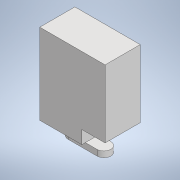
# Autodesk Inventor part: servo
Saved by Autodesk Inventor 2020 (Build 240168000, 168)
## iProperties
Created: 2022-02-17
Part Number: servo
Material: Generic
Document SubType Name: Modeling
Designer: rwte
Density: 1 g/cm^3
Appearance: Default
Author: rwte
Autodesk Inventor part; units mm, degrees
ref_plane "YZ Plane" through (0, 0, 0) normal (1, 0, 0) x (0, 1, 0)
ref_plane "XZ Plane" through (0, 0, 0) normal (0, 1, 0) x (-1, 0, 0)
ref_plane "XY Plane" through (0, 0, 0) normal (0, 0, 1) x (1, 0, 0)
sketch "Sketch1" plane through (0, 0, 0) normal (0, 0, 1) x (1, 0, 0)
  line L0 (0, 0) -> (22.5, 0)
  line L1 (22.5, 0) -> (22.5, 23.3)
  line L2 (22.5, 23.3) -> (0, 23.3)
  line L3 (0, 23.3) -> (0, 0)
  line L4 (0, 0) -> (14.5, 0)
  line L5 (14.5, 0) -> (14.5, -4.5)
  line L6 (0, -4.5) -> (0, 0)
  line L7 (0, -4.5) -> (14.5, -4.5)
  dimension "d0" = 23.3
  dimension "d1" = 22.5
  dimension "d2" = 14.5
  dimension "d3" = 4.5
  constraints: 16 end point, 3 parallel, 2 horizontal, 2 perpendicular, 1 point on line
  measures "d0" distance of L0.end L1.end
  measures "d1" distance of L1.end L2.end
  measures "d2" distance between parallel lines of L6 L5
  measures "d3" distance of L4.end L5.end
extrude "Extrusion1" add sketch "Sketch1" along normal blind 12.1
sketch "Sketch2" plane through (0, -4.5, 0) normal (0, -1, 0) x (1, 0, 0)
  line L0 (0, 0) -> (14.5, 0) projected
  line L1 (14.5, 0) -> (14.5, 12.1) projected
  line L2 (0, 12.1) -> (14.5, 12.1) projected
  line L3 (0, 0) -> (0, 12.1) projected
  line L4 (0, 0) -> (0, 12.1) projected
  line L5 (0, 6.05) -> (14.5, 6.05) construction
  line L6 (0, 12.1) -> (14.5, 12.1) projected
  line L7 (0, 0) -> (14.5, 0) projected
  circle A0 centre (6.05, 6.05) radius 6.05 construction
  line L8 (6.05, 6.05) -> (6.05, 0) construction
  circle A1 centre (6.05, 6.05) radius 2.35
  dimension "d6" = 4.7
  constraints: 4 end point, 2 midpoint, 2 point on line, 1 centre point, 1 coincident, 1 horizontal, 1 vertical, 1 vertical alignment, 2 other
  measures "d6" diameter of A1
extrude "Extrusion2" add sketch "Sketch2" along normal blind 4.5 contours A1
sketch "Sketch3" plane through (6.05, -9, 6.05) normal (0, -1, 0) x (1, 0, 0)
  line L0 (0, 0) -> (10, 0) construction
  line L1 (0, -2.35) -> (10, -2.35)
  line L2 (10, 2.35) -> (0, 2.35)
  arc A0 (0, 2.35) -> (0, -2.35) centre (0, 0) ccw
  arc A1 (10, -2.35) -> (10, 2.35) centre (10, 0) ccw
  circle A2 centre (0, 0) radius 2.35 projected
  point P0 (-6.05, -6.05)
  point P1 (5, 0)
  point P2 (-2.35, 0)
  dimension "d9" = 10
  constraints: 8 end point, 5 point on circle, 4 tangent, 2 centre point, 1 coincident, 1 horizontal, 1 horizontal alignment, 1 midpoint, 1 parallel, 1 other
  measures "d9" distance of L0.end L0.start
extrude "Extrusion3" add sketch "Sketch3" against normal blind 2
body "Solid1"
